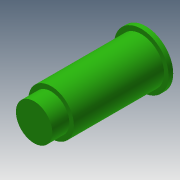
# Autodesk Inventor part: Button
Saved by Autodesk Inventor 2014 (Build 180170000, 170)
## iProperties
Created: 2015-02-17
Part Number: Button
Material: Generic
Document SubType Name: Modeling
Designer: Peele
Density: 1 g/cm^3
Appearance: Default
Author: Peele
Autodesk Inventor part; units mm, degrees
ref_plane "YZ Plane" through (0, 0, 0) normal (1, 0, 0) x (0, 1, 0)
ref_plane "XZ Plane" through (0, 0, 0) normal (0, 1, 0) x (-1, 0, 0)
ref_plane "XY Plane" through (0, 0, 0) normal (0, 0, 1) x (1, 0, 0)
sketch "Sketch1" plane through (0, 0, 0) normal (0, 0, 1) x (1, 0, 0)
  line L0 (0, 0) -> (9, 0)
  line L1 (9, 0) -> (9, -1.5)
  line L2 (9, -1.5) -> (7.5, -1.5)
  line L3 (7.5, -1.5) -> (7.5, -31.2)
  line L4 (7.5, -31.2) -> (6, -31.2)
  line L5 (6, -31.2) -> (6, -36.8)
  line L6 (6, -36.8) -> (0, -36.8)
  line L7 (0, -36.8) -> (0, 0)
  dimension "d0" = 9
  dimension "d1" = 1.5
  dimension "d2" = 29.7
  dimension "d3" = 5.6
  dimension "d4" = 7.5
  dimension "d5" = 6
  constraints: 16 end point, 5 parallel, 2 perpendicular, 1 horizontal
  measures "d0" distance of L0.start L0.end
  measures "d1" distance of L0.end L1.end
  measures "d2" distance of L2.end L3.end
  measures "d3" distance of L4.end L5.end
  measures "d4" distance between parallel lines of L7 L3
  measures "d5" distance of L5.end L6.end
revolve "Revolution1" add sketch "Sketch1" angle 360 about axis through (0, -36.8, 0) along (0, 1, 0)
body "Solid1"
